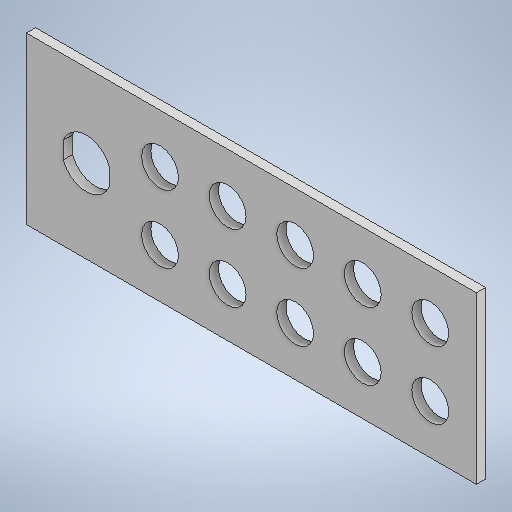
# Autodesk Inventor part: button-front
Saved by Autodesk Inventor 2025.2 (Build 292293000, 293)
## iProperties
Created: 2025-04-18
Part Number: button-front
Material: Generic
Document SubType Name: Modeling
Designer: tdeboutte
Density: 1 g/cm^3
Appearance: Default
Author: tdeboutte
Autodesk Inventor part; units mm, degrees
ref_plane "YZ Plane" through (0, 0, 0) normal (1, 0, 0) x (0, 1, 0)
ref_plane "XZ Plane" through (0, 0, 0) normal (0, 1, 0) x (-1, 0, 0)
ref_plane "XY Plane" through (0, 0, 0) normal (0, 0, 1) x (1, 0, 0)
sketch "Sketch1" plane through (0, 0, 0) normal (0, 0, 1) x (1, 0, 0)
  line L0 (0, 0) -> (146.5, 0)
  line L1 (146.5, 0) -> (146.5, 54)
  line L2 (146.5, 54) -> (0, 54)
  line L3 (0, 54) -> (0, 0)
  circle A0 centre (43.5, 16) radius 6
  circle A1 centre (65.5, 16) radius 6
  circle A2 centre (87.5, 16) radius 6
  circle A3 centre (109.5, 16) radius 6
  circle A4 centre (131.5, 16) radius 6
  circle A5 centre (43.5, 38) radius 6
  circle A6 centre (65.5, 38) radius 6
  circle A7 centre (87.5, 38) radius 6
  circle A8 centre (109.5, 38) radius 6
  circle A9 centre (131.5, 38) radius 6
  circle A10 centre (19.5, 27) radius 8
  line L4 (27, 19) -> (12, 19)
  line L5 (12, 19) -> (12, 35)
  line L6 (12, 35) -> (27, 35)
  line L7 (27, 35) -> (27, 19)
  line L8 (27, 19) -> (12, 35) construction
  line L9 (12, 19) -> (27, 35) construction
  point P0 (27, 24.2161)
  point P1 (12, 24.2161)
  point P2 (12, 29.7839)
  point P3 (27, 29.7839)
  dimension "d0" = 12
  dimension "d3" = 22
  dimension "d6" = 22
  dimension "d9" = 16
  dimension "d10" = 16
  dimension "d11" = 15
  dimension "d12" = 16
  dimension "d13" = 15
  dimension "d14" = 24
  dimension "d15" = 19.5
  dimension "d16" = 67
  dimension "d17" = 27
  constraints: 20 end point, 11 centre point, 4 parallel, 3 horizontal, 2 midpoint, 2 perpendicular, 1 vertical, 18 other
  measures "d0" diameter of A0
  measures "d3" distance of A0.centre A1.centre
  measures "d6" distance of A0.centre A5.centre
  measures "d9" distance from line of L2 A9.centre
  measures "d10" distance from line of L0 A4.centre
  measures "d11" distance from line of L1 A4.centre
  measures "d12" diameter of A10
  measures "d13" distance of L5.end L6.end
  measures "d14" horizontal distance of A5.centre A10.centre
  measures "d15" distance from line of L3 A10.centre
  measures "d17" distance from line of L0 A10.centre
extrude "Extrusion1" add sketch "Sketch1" along normal blind 3 contours L3 L2 L1 L0 | A10 L7 | A10 L6 L7 | L7 L4 A10 | A10 L5 L6 | L4 L5 A10 | L5 A10
body "Solid1"
